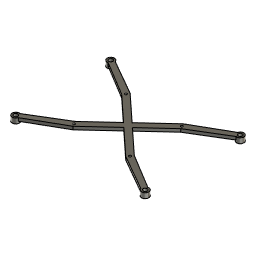
EmlaSafe - PCB Holder (Autodesk Fusion 360 design; units mm, degrees)
Autodesk Fusion 360 part; units mm, degrees
sketch "Sketch1" plane through (0, 0, 0) normal (0, 0, 1) x (1, 0, 0)
  line L0 (0, 0) -> (126.2, 0) construction
  line L1 (126.2, 0) -> (126.2, 92.7) construction
  line L2 (126.2, 92.7) -> (0, 92.7) construction
  line L3 (0, 92.7) -> (0, 0) construction
  circle A0 centre (126.2, 0) radius 2
  circle A1 centre (126.2, 92.7) radius 2
  circle A2 centre (0, 92.7) radius 2
  circle A3 centre (0, 0) radius 2
  line L4 (0, 92.7) -> (-5, 92.7) construction
  line L5 (0, 92.7) -> (0, 97.7) construction
  line L6 (0, 97.7) -> (-5, 92.7) construction
  line L7 (126.2, 0) -> (131.2, 0) construction
  line L8 (126.2, 0) -> (126.2, -5) construction
  line L9 (126.2, -5) -> (131.2, 0) construction
  line L10 (-2.5, 95.2) -> (128.7, 95.2)
  line L11 (128.7, 95.2) -> (128.7, -2.5)
  line L12 (128.7, -2.5) -> (-2.5, -2.5)
  line L13 (-2.5, -2.5) -> (-2.5, 95.2)
  line L14 (35.8499, 71.5999) -> (90.3499, 71.5999) construction
  line L15 (90.3499, 71.5999) -> (90.3499, 21.0999) construction
  line L16 (90.3499, 21.0999) -> (35.8499, 21.0999) construction
  line L17 (35.8499, 21.0999) -> (35.8499, 71.5999) construction
  line L18 (126.2, 0) -> (0, 92.7) construction
  line L19 (126.2, 92.7) -> (0, 0) construction
  line L20 (35.8499, 71.5999) -> (90.3499, 21.0999) construction
  line L21 (90.3499, 71.5999) -> (35.8499, 21.0999) construction
  circle A4 centre (35.8499, 71.5999) radius 1.3
  circle A5 centre (90.3499, 71.5999) radius 1.3
  circle A6 centre (90.3499, 21.0999) radius 1.3
  circle A7 centre (35.8499, 21.0999) radius 1.3
  circle A8 centre (90.3499, 71.5999) radius 3
  circle A9 centre (35.8499, 71.5999) radius 3
  circle A10 centre (35.8499, 21.0999) radius 3
  circle A11 centre (90.3499, 21.0999) radius 3
  circle A12 centre (126.2, 0) radius 2.5
  circle A13 centre (126.2, 92.7) radius 2.5
  circle A14 centre (0, 92.7) radius 2.5
  circle A15 centre (0, 0) radius 2.5
  line L22 (-1.5, 2) -> (34.2965, 23.6664)
  line L23 (1.5, -2) -> (37.3392, 18.4957)
  line L24 (91.9033, 23.6664) -> (127.4939, 2.1391)
  line L25 (88.8606, 18.4957) -> (124.7009, -2.0006)
  line L26 (37.3392, 74.2041) -> (1.5012, 94.6991)
  line L27 (34.2965, 69.0334) -> (-1.2939, 90.5609)
  line L28 (91.9033, 69.0334) -> (127.4939, 90.5609)
  line L29 (88.8606, 74.2041) -> (124.6996, 94.6997)
  line L30 (37.3392, 18.4957) -> (91.9033, 69.0334)
  line L31 (34.2965, 23.6664) -> (88.8606, 74.2041)
  line L32 (34.2965, 69.0334) -> (88.309, 18.9011)
  line L33 (91.9033, 23.6664) -> (37.3392, 74.2041)
  circle A16 centre (0, 92.7) radius 3.5
  circle A17 centre (0, 0) radius 3.5
  circle A18 centre (126.2, 0) radius 3.5
  circle A19 centre (126.2, 92.7) radius 3.5
  point P0 (-2.5, 95.2)
  point P1 (128.7, -2.5)
  dimension "d1" = 126.2
  dimension "d2" = 92.7
  dimension "d3" = 4
  dimension "d4" = 4
  dimension "d5" = 4
  dimension "d6" = 4
  dimension "d7" = 5
  dimension "d8" = 5
  dimension "d9" = 5
  dimension "d10" = 5
  dimension "d11" = 54.5
  dimension "d12" = 50.5
  dimension "d13" = 2.6
  dimension "d14" = 2.6
  dimension "d15" = 2.6
  dimension "d16" = 2.6
  dimension "d17" = 6
  dimension "d18" = 6
  dimension "d19" = 6
  dimension "d20" = 6
  dimension "d25" = 7
  dimension "d26" = 7
  dimension "d27" = 7
  dimension "d28" = 7
  constraint horizontal L0
  constraint vertical L1
  constraint horizontal L2
  constraint vertical L3
  constraint coincident L0.start L3.end
  constraint coincident L0.end L1.start
  constraint coincident L1.end L2.start
  constraint coincident L2.end L3.start
  constraint perpendicular L3 L4
  constraint perpendicular L4 L5
  constraint midpoint L6 P0
  constraint perpendicular L1 L7
  constraint perpendicular L0 L8
  constraint midpoint L9 P1
  constraint horizontal L10
  constraint vertical L11
  constraint horizontal L12
  constraint vertical L13
  constraint coincident P1 L11.end
  constraint coincident P0 L10.start
  constraint horizontal L14
  constraint vertical L15
  constraint horizontal L16
  constraint vertical L17
  constraint coincident L14.start L17.end
  constraint coincident L14.end L15.start
  constraint coincident L15.end L16.start
  constraint coincident L16.end L17.start
  constraint concentric A5 A8
  constraint concentric A4 A9
  constraint concentric A7 A10
  constraint concentric A6 A11
  constraint concentric A0 A12
  constraint tangent L11 A12
  constraint concentric A1 A13
  constraint tangent L10 A13
  constraint concentric A2 A14
  constraint tangent L13 A15
  constraint coincident A15 L22.start
  constraint coincident A10 L22.end
  constraint tangent A10 L22
  constraint coincident A15 L23.start
  constraint coincident A10 L23.end
  constraint tangent A10 L23
  constraint coincident A11 L24.start
  constraint coincident A12 L24.end
  constraint tangent A12 L24
  constraint coincident A11 L25.start
  constraint coincident A12 L25.end
  constraint tangent A11 L25
  constraint coincident A9 L26.start
  constraint coincident A14 L26.end
  constraint tangent A9 L26
  constraint parallel L25 L26
  constraint coincident A9 L27.start
  constraint coincident A14 L27.end
  constraint tangent A14 L27
  constraint coincident A8 L28.start
  constraint coincident A13 L28.end
  constraint tangent A13 L28
  constraint coincident A8 L29.start
  constraint coincident A13 L29.end
  constraint tangent A8 L29
  constraint parallel L30 L31
  constraint coincident A11 L32.end
  constraint tangent A11 L32
  constraint concentric A2 A16
  constraint concentric A0 A18
  constraint concentric A1 A19
  measures "d1" distance of L0.start L0.end
  measures "d2" distance of L0.start L2.end
  measures "d3" diameter of A0
  measures "d4" diameter of A1
  measures "d5" diameter of A2
  measures "d6" diameter of A3
  measures "d7" distance of L2.end L4.end
  measures "d8" distance of L2.end L5.end
  measures "d9" distance of L0.end L7.end
  measures "d10" distance of L0.end L8.end
  measures "d11" distance of L14.start L14.end
  measures "d12" distance of L14.start L16.end
  measures "d13" diameter of A4
  measures "d14" diameter of A5
  measures "d15" diameter of A6
  measures "d16" diameter of A7
  measures "d17" diameter of A8
  measures "d18" diameter of A9
  measures "d19" diameter of A10
  measures "d20" diameter of A11
  measures "d25" diameter of A16
  measures "d26" diameter of A17
  measures "d27" diameter of A18
  measures "d28" diameter of A19
extrude "Extrude1" add sketch "Sketch1" along normal blind 3 contours A14 | A14 L26 L27 A16 | A9 L26 L27 A16 | A13 | A8 L28 L29 A19 | A13 L28 L29 A19 | A9 L33 | A15 L22 | A15 L22 L23 A17 | A10 L22 L23 A17 | A9 L31 L32 L33 | A8 L31 | A10 L30 L31 L32 | A10 L30 | L30 L31 L32 L33 | A8 L30 L31 L33 | A11 L30 L32 L33 | A11 | A12 | A11 L24 L25 A18 | A12 L24 L25 A18 picked at (37.444, 73.3682) picked at (-1.1921, 1.9962) picked at (88.7557, 73.3682) picked at (37.444, 19.3316)
extrude "Extrude2" add sketch "Sketch1" along normal blind -2 and the other way blind -3 contours L10 A16 | L10 L13 A14 A16 | L13 A16 | L10 A14 L26 A16 | A14 | L13 A14 L27 A16 | A14 L26 L27 A16 | L10 A19 | L10 A13 L29 A19 | L13 A15 L22 A17 | L13 A17 | L10 L11 A13 A19 | A13 | A13 L28 L29 A19 | L12 L13 A15 A17 | A15 L22 | A15 L22 L23 A17 | L11 A19 | L11 A13 L28 A19 | L12 A15 L23 A17 | L12 A17 | L11 A18 | L11 A12 L24 A18 | L12 A12 L25 A18 | L12 A18 | A12 | L11 L12 A12 A18 | A12 L24 L25 A18 picked at (-1.1921, 1.9962)
thread "Thread1" "ISO Metric profile 2.5 M2.5x0.45 6H" major diameter 2.58 minor diameter 2.0755 pitch 0.45 angle 60 resizes the face on face at (90.3823, 72.8995, 2) on face at (36.9591, 72.2778, 2) on face at (35.4358, 22.3322, 2) on face at (90.3823, 22.3995, 2)
